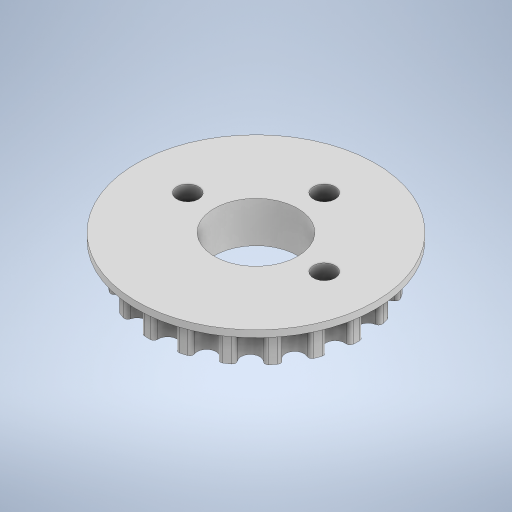
# Autodesk Inventor part: 射出_プーリ_歯数20
Saved by Autodesk Inventor 2023 (Build 270158000, 158)
## iProperties
Created: 2022-04-22
Part Number: 射出_プーリ_歯数20
Material: 一般
Document SubType Name: Modeling
Designer: yuta
Density: 1 g/cm^3
Appearance: 既定
Author: yuta
Autodesk Inventor part; units mm, degrees
ref_plane "YZ Plane" through (0, 0, 0) normal (1, 0, 0) x (0, 1, 0)
ref_plane "XZ Plane" through (0, 0, 0) normal (0, 1, 0) x (-1, 0, 0)
ref_plane "XY Plane" through (0, 0, 0) normal (0, 0, 1) x (1, 0, 0)
sketch "スケッチ1" plane through (0, 0, 0) normal (0, 1, 0) x (-1, 0, 0)
  circle A0 centre (0, 0) radius 15.915 construction
  arc A1 (15.3064, -1.0659) -> (15.3428, -0.1435) centre (0, 0) ccw construction
  circle A2 centre (0, 0) radius 13.4135 construction
  line L0 (0, 0) -> (13.3208, 1.5743)
  line L1 (0, 0) -> (13.1553, -2.6191)
  arc A3 (13.3208, 1.5743) -> (14.7917, 0.3696) centre (14.6813, 1.7351) ccw
  arc A4 (14.7166, -1.534) -> (15.3064, -1.0659) centre (14.7977, -1.0305) ccw
  arc A5 (14.7166, -1.534) -> (13.1553, -2.6191) centre (14.499, -2.8866) ccw
  arc A6 (15.3428, -0.1435) -> (14.7917, 0.3696) centre (14.8329, -0.1388) ccw
  arc A7 (15.3428, -0.1435) -> (15.3064, -1.0659) centre (0, 0) ccw construction
  arc A8 (15.3064, -1.0659) -> (15.3428, -0.1435) centre (0, 0) ccw
  dimension "d0" = 31.83
  dimension "d2" = 26.827
  dimension "d3" = 18
  constraints: 16 point on circle, 9 centre point, 4 coincident, 4 end point, 1 tangent
  measures "d0" diameter of A0
  measures "d2" diameter of A2
  measures "d3" angle of L1 L0
extrude "押し出し1" add sketch "スケッチ1" along normal blind 5
pattern_circular "円形状パターン1" count 20 over 360 about axis through (0, 0, 0) along (0, 1, 0) of "押し出し1"
sketch "スケッチ2" plane through (0, 5, 0) normal (0, 1, 0) x (1, 0, 0)
  circle A0 centre (0, 0) radius 16
  dimension "d13" = 32
  constraints: 1 centre point, 1 coincident
  measures "d13" diameter of A0
extrude "押し出し2" add sketch "スケッチ2" along normal blind 1
sketch "スケッチ3" plane through (0, 0, 0) normal (0, -1, 0) x (1, 0, 0)
  circle A0 centre (0, 0) radius 6
  circle A1 centre (0, -10) radius 1.6
  circle A2 centre (-10, 0) radius 1.6
  circle A3 centre (10, 0) radius 1.6
  dimension "d16" = 12
  dimension "d17" = 3.2
  dimension "d18" = 10
  dimension "d19" = 3.2
  dimension "d20" = 3.2
  dimension "d21" = 10
  dimension "d22" = 10
  constraints: 4 centre point, 1 coincident
  measures "d16" diameter of A0
  measures "d17" diameter of A1
  measures "d18" distance of point (0, 0) A1.centre
  measures "d19" diameter of A2
  measures "d20" diameter of A3
  measures "d21" distance of point (0, 0) A2.centre
  measures "d22" distance of point (0, 0) A3.centre
extrude "押し出し3" cut sketch "スケッチ3" against normal blind 6
sketch "スケッチ4" plane through (0, 0, 0) normal (0, -1, 0) x (1, 0, 0)
  point P0 (0, 0)
sketch "スケッチ5" plane through (0, 0, 0) normal (0, -1, 0) x (1, 0, 0)
  circle A0 centre (0, 0) radius 6.1
  dimension "d25" = 12.2
  constraints: 1 centre point, 1 coincident
  measures "d25" diameter of A0
extrude "押し出し4" cut sketch "スケッチ5" against normal blind 6
sketch "スケッチ6" plane through (0, 6, 0) normal (0, 1, 0) x (1, 0, 0)
  circle A0 centre (0, 0) radius 17.5
  circle A1 centre (0, 0) radius 16
  circle A2 centre (0, 0) radius 16
  dimension "d28" = 35
  constraints: 3 centre point, 3 coincident, 1 concentric
  measures "d28" diameter of A0
extrude "押し出し5" add sketch "スケッチ6" against normal blind 1
